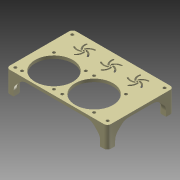
# Autodesk Inventor part: Tapa carcasa SAV
Saved by Autodesk Inventor 2014 (Build 180170000, 170)
## iProperties
Created: 2014-09-11
Part Number: Tapa carcasa SAV
Material: Nylon, molybdenum disulphide
Document SubType Name: Modeling
Designer: Rubén
Density: 1.13 g/cm^3
Appearance: Nylon 6
Mass: 26.3943 g
Surface Area: 167.072 cm^2
Volume: 23.3578 cm^3
Author: Rubén
Autodesk Inventor part; units mm, degrees
ref_plane "YZ Plane" through (0, 0, 0) normal (1, 0, 0) x (0, 1, 0)
ref_plane "XZ Plane" through (0, 0, 0) normal (0, 1, 0) x (-1, 0, 0)
ref_plane "XY Plane" through (0, 0, 0) normal (0, 0, 1) x (1, 0, 0)
sketch "Sketch1" plane through (0, 0, 0) normal (0, 1, 0) x (-1, 0, 0)
  line L0 (6.59, 3) -> (101.11, 3)
  line L1 (104.7, 6.59) -> (104.7, 66.18)
  line L2 (101.11, 69.77) -> (6.59, 69.77)
  line L3 (3, 66.18) -> (3, 6.59)
  arc A0 (6.59, 69.77) -> (3, 66.18) centre (6.59, 66.18) ccw
  arc A1 (104.7, 66.18) -> (101.11, 69.77) centre (101.11, 66.18) ccw
  arc A2 (101.11, 3) -> (104.7, 6.59) centre (101.11, 6.59) ccw
  arc A3 (3, 6.59) -> (6.59, 3) centre (6.59, 6.59) ccw
  line L4 (61.1, 41.9) -> (61.1, 62.5) construction
  line L5 (61.1, 41.9) -> (97.35, 41.9) construction
  line L6 (61.1, 41.9) -> (24.85, 41.9) construction
  line L7 (24.85, 41.9) -> (24.85, 62.5) construction
  line L8 (24.85, 62.5) -> (97.35, 62.5) construction
  line L9 (97.35, 62.5) -> (97.35, 41.9) construction
  line L10 (61.8884, 68.7185) -> (93.8884, 68.7185) construction
  line L11 (98.0634, 64.5435) -> (98.0634, 32.5435) construction
  line L12 (93.8884, 28.3685) -> (61.8884, 28.3685) construction
  line L13 (57.7134, 32.5435) -> (57.7134, 64.5435) construction
  line L14 (53.5384, 68.7185) -> (21.5384, 68.7185) construction
  line L15 (17.3634, 64.5435) -> (17.3634, 32.5435) construction
  line L16 (21.5384, 28.3685) -> (53.5384, 28.3685) construction
  circle A4 centre (21.538, 32.544) radius 1.5
  arc A5 (21.5384, 68.7185) -> (17.3634, 64.5435) centre (21.5384, 64.5435) ccw construction
  arc A6 (17.3634, 32.5435) -> (21.5384, 28.3685) centre (21.5384, 32.5435) ccw construction
  arc A7 (53.5384, 28.3685) -> (57.7134, 32.5435) centre (53.5384, 32.5435) ccw construction
  arc A8 (57.7134, 32.5435) -> (61.8884, 28.3685) centre (61.8884, 32.5435) ccw construction
  arc A9 (93.8884, 28.3685) -> (98.0634, 32.5435) centre (93.8884, 32.5435) ccw construction
  arc A10 (98.0634, 64.5435) -> (93.8884, 68.7185) centre (93.8884, 64.5435) ccw construction
  arc A11 (57.7134, 64.5435) -> (53.5384, 68.7185) centre (53.5384, 64.5435) ccw construction
  arc A12 (61.8884, 68.7185) -> (57.7134, 64.5435) centre (61.8884, 64.5435) ccw construction
  circle A13 centre (21.5384, 64.5435) radius 1.5
  circle A14 centre (61.8884, 64.5435) radius 1.5
  circle A15 centre (53.5384, 64.5435) radius 1.5
  circle A16 centre (93.8884, 64.5435) radius 1.5
  circle A17 centre (61.8884, 32.5435) radius 1.5
  circle A18 centre (53.5384, 32.5435) radius 1.5
  circle A19 centre (93.8884, 32.5435) radius 1.5
  circle A20 centre (37.5384, 48.5435) radius 19
  circle A21 centre (77.8884, 48.5435) radius 19
  circle A22 centre (53.85, 15.8218) radius 0.75
  arc A23 (58.578, 8.7134) -> (56.37, 16.3622) centre (50.85, 10.6256) ccw
  arc A24 (57.122, 9.0737) -> (55.33, 15.2814) centre (50.85, 10.6256) ccw
  arc A25 (57.122, 9.0737) -> (58.578, 8.7134) centre (57.85, 8.8936) ccw
  arc A26 (56.37, 16.3622) -> (55.33, 15.2814) centre (55.85, 15.8218) ccw
  circle A27 centre (80.75, 15.8218) radius 0.75
  arc A28 (85.478, 8.7134) -> (83.27, 16.3622) centre (77.75, 10.6256) ccw
  arc A29 (84.022, 9.0737) -> (82.23, 15.2814) centre (77.75, 10.6256) ccw
  arc A30 (84.022, 9.0737) -> (85.478, 8.7134) centre (84.75, 8.8936) ccw
  arc A31 (83.27, 16.3622) -> (82.23, 15.2814) centre (82.75, 15.8218) ccw
  arc A32 (88.9715, 18.1218) -> (81.0148, 18.3855) centre (84.7648, 11.3629) ccw
  arc A33 (88.1789, 16.8483) -> (81.7213, 17.0623) centre (84.7648, 11.3629) ccw
  arc A34 (81.0148, 18.3855) -> (81.7213, 17.0623) centre (81.368, 17.7239) ccw
  arc A35 (88.1789, 16.8483) -> (88.9715, 18.1218) centre (88.5752, 17.4851) ccw
  arc A36 (81.1031, 24.3516) -> (78.3936, 16.8658) centre (86.2313, 18.2622) ccw
  arc A37 (82.0693, 23.2043) -> (79.8703, 17.1289) centre (86.2313, 18.2622) ccw
  arc A38 (78.3936, 16.8658) -> (79.8703, 17.1289) centre (79.132, 16.9974) ccw
  arc A39 (82.0693, 23.2043) -> (81.1031, 24.3516) centre (81.5862, 23.778) ccw
  arc A40 (72.7468, 18.7935) -> (79.0289, 13.9033) centre (80.1228, 21.7889) ccw
  arc A41 (74.1365, 19.3579) -> (79.235, 15.3891) centre (80.1228, 21.7889) ccw
  arc A42 (79.0289, 13.9033) -> (79.235, 15.3891) centre (79.132, 14.6462) ccw
  arc A43 (74.1365, 19.3579) -> (72.7468, 18.7935) centre (73.4416, 19.0757) ccw
  arc A44 (75.4506, 9.1285) -> (82.0427, 13.5921) centre (74.8811, 17.0693) ccw
  arc A45 (75.3433, 10.6247) -> (80.6934, 14.2473) centre (74.8811, 17.0693) ccw
  arc A46 (82.0427, 13.5921) -> (80.6934, 14.2473) centre (81.368, 13.9197) ccw
  arc A47 (75.3433, 10.6247) -> (75.4506, 9.1285) centre (75.397, 9.8766) ccw
  circle A48 centre (26.95, 15.8218) radius 0.75
  arc A49 (31.678, 8.7134) -> (29.47, 16.3622) centre (23.95, 10.6256) ccw
  arc A50 (30.222, 9.0737) -> (28.43, 15.2814) centre (23.95, 10.6256) ccw
  arc A51 (30.222, 9.0737) -> (31.678, 8.7134) centre (30.95, 8.8936) ccw
  arc A52 (29.47, 16.3622) -> (28.43, 15.2814) centre (28.95, 15.8218) ccw
  arc A53 (35.1715, 18.1218) -> (27.2148, 18.3855) centre (30.9648, 11.3629) ccw
  arc A54 (34.3789, 16.8483) -> (27.9213, 17.0623) centre (30.9648, 11.3629) ccw
  arc A55 (27.2148, 18.3855) -> (27.9213, 17.0623) centre (27.568, 17.7239) ccw
  arc A56 (34.3789, 16.8483) -> (35.1715, 18.1218) centre (34.7752, 17.4851) ccw
  arc A57 (27.3031, 24.3516) -> (24.5936, 16.8658) centre (32.4313, 18.2622) ccw
  arc A58 (28.2693, 23.2043) -> (26.0703, 17.1289) centre (32.4313, 18.2622) ccw
  arc A59 (24.5936, 16.8658) -> (26.0703, 17.1289) centre (25.332, 16.9974) ccw
  arc A60 (28.2693, 23.2043) -> (27.3031, 24.3516) centre (27.7862, 23.778) ccw
  arc A61 (18.9468, 18.7935) -> (25.2289, 13.9033) centre (26.3228, 21.7889) ccw
  arc A62 (20.3365, 19.3579) -> (25.435, 15.3891) centre (26.3228, 21.7889) ccw
  arc A63 (25.2289, 13.9033) -> (25.435, 15.3891) centre (25.332, 14.6462) ccw
  arc A64 (20.3365, 19.3579) -> (18.9468, 18.7935) centre (19.6416, 19.0757) ccw
  arc A65 (21.6506, 9.1285) -> (28.2427, 13.5921) centre (21.0811, 17.0693) ccw
  arc A66 (21.5433, 10.6247) -> (26.8934, 14.2473) centre (21.0811, 17.0693) ccw
  arc A67 (28.2427, 13.5921) -> (26.8934, 14.2473) centre (27.568, 13.9197) ccw
  arc A68 (21.5433, 10.6247) -> (21.6506, 9.1285) centre (21.597, 9.8766) ccw
  circle A69 centre (53.85, 15.8218) radius 0.75
  arc A70 (58.578, 8.7134) -> (56.37, 16.3622) centre (50.85, 10.6256) ccw
  arc A71 (57.122, 9.0737) -> (55.33, 15.2814) centre (50.85, 10.6256) ccw
  arc A72 (57.122, 9.0737) -> (58.578, 8.7134) centre (57.85, 8.8936) ccw
  arc A73 (56.37, 16.3622) -> (55.33, 15.2814) centre (55.85, 15.8218) ccw
  arc A74 (62.0715, 18.1218) -> (54.1148, 18.3855) centre (57.8648, 11.3629) ccw
  arc A75 (61.2789, 16.8483) -> (54.8213, 17.0623) centre (57.8648, 11.3629) ccw
  arc A76 (54.1148, 18.3855) -> (54.8213, 17.0623) centre (54.468, 17.7239) ccw
  arc A77 (61.2789, 16.8483) -> (62.0715, 18.1218) centre (61.6752, 17.4851) ccw
  arc A78 (54.2031, 24.3516) -> (51.4936, 16.8658) centre (59.3313, 18.2622) ccw
  arc A79 (55.1693, 23.2043) -> (52.9703, 17.1289) centre (59.3313, 18.2622) ccw
  arc A80 (51.4936, 16.8658) -> (52.9703, 17.1289) centre (52.232, 16.9974) ccw
  arc A81 (55.1693, 23.2043) -> (54.2031, 24.3516) centre (54.6862, 23.778) ccw
  arc A82 (45.8468, 18.7935) -> (52.1289, 13.9033) centre (53.2228, 21.7889) ccw
  arc A83 (47.2365, 19.3579) -> (52.335, 15.3891) centre (53.2228, 21.7889) ccw
  arc A84 (52.1289, 13.9033) -> (52.335, 15.3891) centre (52.232, 14.6462) ccw
  arc A85 (47.2365, 19.3579) -> (45.8468, 18.7935) centre (46.5416, 19.0757) ccw
  arc A86 (48.5506, 9.1285) -> (55.1427, 13.5921) centre (47.9811, 17.0693) ccw
  arc A87 (48.4433, 10.6247) -> (53.7934, 14.2473) centre (47.9811, 17.0693) ccw
  arc A88 (55.1427, 13.5921) -> (53.7934, 14.2473) centre (54.468, 13.9197) ccw
  arc A89 (48.4433, 10.6247) -> (48.5506, 9.1285) centre (48.497, 9.8766) ccw
  circle A90 centre (7.495, 64.96) radius 1.5
  circle A91 centre (7.495, 7.81) radius 1.5
  circle A92 centre (100.205, 7.81) radius 1.5
  circle A93 centre (100.205, 64.96) radius 1.5
  line L17 (3, 36.385) -> (104.7, 36.385) construction
  line L18 (53.85, 3) -> (53.85, 69.77) construction
  point P0 (0, 0)
  point P1 (3, 3)
  point P2 (104.7, 3)
  point P3 (104.7, 69.77)
  point P4 (3, 69.77)
  point P5 (57.7134, 68.7185)
  point P6 (98.0634, 28.3685)
  point P7 (98.0634, 68.7185)
  point P8 (57.7134, 28.3685)
  point P9 (17.3634, 68.7185)
  point P10 (17.3634, 28.3685)
  point P11 (61.6752, 17.4851)
  point P12 (61.2789, 16.8483)
  point P13 (54.8213, 17.0623)
  point P14 (52.232, 16.9974)
  point P15 (59.3313, 18.2622)
  point P16 (52.9703, 17.1289)
  point P17 (45.8468, 18.7935)
  point P18 (47.2365, 19.3579)
  point P19 (52.1289, 13.9033)
  point P20 (48.497, 9.8766)
  point P21 (48.4433, 10.6247)
  point P22 (53.7934, 14.2473)
  dimension "d2" = 101.7
  dimension "d3" = 66.77
  dimension "d4" = 101.7
  dimension "d5" = 3.59
  dimension "d6" = 3.59
  dimension "d21" = 36.25
  dimension "d22" = 36.25
  dimension "d23" = 20.6
  dimension "d24" = 40.35
  dimension "d25" = 40.35
  dimension "d26" = 40.35
  dimension "d27" = 40.35
  dimension "d28" = 40.35
  dimension "d29" = 3
  dimension "d30" = 4.175
  dimension "d31" = 3
  dimension "d32" = 3
  dimension "d33" = 3
  dimension "d34" = 3
  dimension "d35" = 3
  dimension "d36" = 3
  dimension "d37" = 3
  dimension "d40" = 38
  dimension "d41" = 38
  dimension "d71" = 26.9
  dimension "d74" = 26.9
  dimension "d83" = 3
  dimension "d84" = 3
  dimension "d85" = 3
  dimension "d86" = 3
  dimension "d192" = 57.15
  dimension "d193" = 28.575
  dimension "d194" = 57.15
  dimension "d195" = 28.575
  dimension "d196" = 92.71
  dimension "d197" = 92.71
  dimension "d198" = 46.355
  dimension "d199" = 46.355
  constraints: 152 point on circle, 94 centre point, 38 end point, 28 tangent, 24 point on line, 9 equal radius, 8 perpendicular, 7 coincident, 5 midpoint, 4 equal length, 3 horizontal
  measures "d2" distance of point (3, 3) point (104.7, 3)
  measures "d3" distance of point (104.7, 3) point (104.7, 69.77)
  measures "d4" distance of point (104.7, 69.77) point (3, 69.77)
  measures "d5" radius of A0
  measures "d6" radius of A1
  measures "d21" distance of L4.start L5.end
  measures "d22" distance of L4.start L6.end
  measures "d23" distance of L6.end L7.end
  measures "d24" distance of point (98.063, 28.369) point (57.713, 28.369)
  measures "d25" distance of point (98.063, 68.719) point (98.063, 28.369)
  measures "d26" distance of point (57.713, 68.719) point (17.363, 68.719)
  measures "d27" distance of point (17.363, 68.719) point (17.363, 28.369)
  measures "d28" distance of point (17.363, 28.369) point (57.713, 28.369)
  measures "d29" diameter of A4
  measures "d30" radius of A5
  measures "d31" diameter of A13
  measures "d32" diameter of A14
  measures "d33" diameter of A15
  measures "d34" diameter of A16
  measures "d35" diameter of A17
  measures "d36" diameter of A18
  measures "d37" diameter of A19
  measures "d40" diameter of A20
  measures "d41" diameter of A21
  measures "d71" distance of point (59.331, 18.262) A36.centre
  measures "d74" distance of point (59.331, 18.262) A57.centre
  measures "d83" diameter of A90
  measures "d84" diameter of A91
  measures "d85" diameter of A92
  measures "d86" diameter of A93
  measures "d192" distance of A91.centre A90.centre
  measures "d193" distance from line of L17 A91.centre
  measures "d194" distance of A93.centre A92.centre
  measures "d195" distance from line of L17 A92.centre
  measures "d196" distance of A93.centre A90.centre
  measures "d197" distance of A92.centre A91.centre
  measures "d198" distance from line of L18 A91.centre
  measures "d199" distance from line of L18 A90.centre
extrude "Extrusion3" add sketch "Sketch1" along normal blind 3
sketch "Sketch5" plane through (0, 0, 0) normal (0, -1, 0) x (1, 0, 0)
  circle A0 centre (-100.205, 64.96) radius 1.5 projected
  circle A1 centre (-100.205, 7.81) radius 1.5 projected
  line L0 (-6.59, 69.77) -> (-101.11, 69.77) projected
  line L1 (-104.7, 66.18) -> (-104.7, 6.59) projected
  line L2 (-101.11, 3) -> (-6.59, 3) projected
  line L3 (-3, 6.59) -> (-3, 66.18) projected
  arc A2 (-101.11, 69.77) -> (-104.7, 66.18) centre (-101.11, 66.18) ccw projected
  arc A3 (-104.7, 6.59) -> (-101.11, 3) centre (-101.11, 6.59) ccw projected
  arc A4 (-6.59, 3) -> (-3, 6.59) centre (-6.59, 6.59) ccw projected
  arc A5 (-3, 66.18) -> (-6.59, 69.77) centre (-6.59, 66.18) ccw projected
  line L4 (-97.205, 69.77) -> (-101.11, 69.77)
  line L5 (-104.7, 10.81) -> (-104.7, 6.59)
  line L6 (-101.11, 3) -> (-97.205, 3)
  line L7 (-10.495, 3) -> (-6.59, 3)
  line L8 (-3, 6.59) -> (-3, 10.81)
  line L9 (-10.495, 69.77) -> (-6.59, 69.77)
  line L10 (-3, 66.18) -> (-3, 61.96)
  arc A6 (-3, 66.18) -> (-6.59, 69.77) centre (-6.59, 66.18) ccw
  arc A7 (-6.59, 3) -> (-3, 6.59) centre (-6.59, 6.59) ccw
  arc A8 (-104.7, 6.59) -> (-101.11, 3) centre (-101.11, 6.59) ccw
  arc A9 (-101.11, 69.77) -> (-104.7, 66.18) centre (-101.11, 66.18) ccw
  circle A10 centre (-7.495, 7.81) radius 1.5
  circle A11 centre (-7.495, 64.96) radius 1.5
  circle A12 centre (-100.205, 7.81) radius 1.5
  circle A13 centre (-100.205, 64.96) radius 1.5
  arc A14 (-97.205, 7.81) -> (-100.205, 10.81) centre (-100.205, 7.81) ccw
  line L11 (-97.205, 7.81) -> (-97.205, 3)
  line L12 (-100.205, 10.81) -> (-104.7, 10.81)
  arc A15 (-100.205, 61.96) -> (-97.205, 64.96) centre (-100.205, 64.96) ccw
  arc A16 (-10.495, 64.96) -> (-7.495, 61.96) centre (-7.495, 64.96) ccw
  arc A17 (-7.495, 10.81) -> (-10.495, 7.81) centre (-7.495, 7.81) ccw
  line L13 (-7.495, 10.81) -> (-3, 10.81)
  line L14 (-10.495, 7.81) -> (-10.495, 3)
  line L15 (-97.205, 64.96) -> (-97.205, 69.77)
  line L16 (-7.495, 61.96) -> (-3, 61.96)
  line L17 (-10.495, 64.96) -> (-10.495, 69.77)
  circle A18 centre (-7.495, 7.81) radius 1.5 projected
  circle A19 centre (-7.495, 64.96) radius 1.5 projected
  line L18 (-100.205, 61.96) -> (-104.7, 61.96)
  line L19 (-104.7, 66.18) -> (-104.7, 61.96)
  point P0 (-3, 63.52)
  point P1 (-9.25, 69.77)
  point P2 (-104.7, 9.25)
  point P3 (-98.45, 3)
  point P4 (-98.45, 69.77)
  point P5 (-3, 9.25)
  point P6 (-9.25, 3)
  dimension "d142" = 3
  dimension "d143" = 3
  dimension "d144" = 3
  dimension "d145" = 3
  dimension "d146" = 6
  dimension "d147" = 6
  dimension "d148" = 6
  dimension "d149" = 6
  constraints: 32 end point, 22 point on circle, 22 point on line, 12 centre point, 12 coincident, 11 perpendicular, 10 tangent, 3 collinear
  measures "d142" diameter of A10
  measures "d143" diameter of A11
  measures "d144" diameter of A12
  measures "d145" diameter of A13
  measures "d146" diameter of A14
  measures "d147" diameter of A15
  measures "d148" diameter of A16
  measures "d149" diameter of A17
extrude "Extrusion6" add sketch "Sketch5" along normal blind 18.4 contours A5 L3 L16 A16 L17 L0 | L15 A15 L18 L1 A2 L0 | L3 A4 L2 L14 A17 L13 | L12 A14 L11 L2 A3 L1
sketch "Sketch6" plane through (-101.11, 3, 69.77) normal (0, 0, 1) x (1, 0, 0)
  line L0 (6.8339, -9.2711) -> (10.1761, -5.9289)
  arc A0 (17.2471, -3) -> (10.1761, -5.9289) centre (17.2471, -13) ccw
  arc A1 (6.8339, -9.2711) -> (3.905, -16.3421) centre (13.905, -16.3421) ccw
  line L1 (3.905, -3) -> (3.905, -16.3421)
  line L2 (3.905, -3) -> (17.2471, -3)
  line L3 (94.52, -21.4) -> (90.615, -21.4) projected
  line L4 (47.42, -3) -> (47.42, -21.4) construction
  line L5 (88.0061, -9.2711) -> (84.6639, -5.9289)
  arc A2 (84.6639, -5.9289) -> (77.5928, -3) centre (77.5928, -13) ccw
  arc A3 (90.935, -16.3421) -> (88.0061, -9.2711) centre (80.935, -16.3421) ccw
  line L6 (90.935, -3) -> (90.935, -16.3421)
  line L7 (90.935, -3) -> (77.5928, -3)
  point P0 (91.86, -21.4)
  point P1 (101.11, -3)
  point P2 (13.105, -3)
  point P3 (94.52, -3)
  point P4 (0, -3)
  point P5 (3.905, -3)
  point P6 (91.63, -21.4)
  point P7 (81.735, -3)
  point P8 (90.935, -3)
  dimension "d94" = 10
  dimension "d95" = 10
  constraints: 14 end point, 9 symmetric about line, 8 point on circle, 4 centre point, 4 tangent, 2 point on line, 1 perpendicular, 2 other
  measures "d94" radius of A0
  measures "d95" radius of A1
extrude "Extrusion7" add sketch "Sketch6" against normal blind 2.8
sketch "Sketch7" plane through (-6.59, 3, 3) normal (0, 0, -1) x (-1, 0, 0)
  line L0 (90.615, -3) -> (3.905, -3) projected
  line L1 (6.8339, -9.2711) -> (10.1761, -5.9289)
  arc A0 (17.2471, -3) -> (10.1761, -5.9289) centre (17.2471, -13) ccw
  arc A1 (6.8339, -9.2711) -> (3.905, -16.3421) centre (13.905, -16.3421) ccw
  line L2 (3.905, -3) -> (3.905, -16.3421)
  line L3 (3.905, -3) -> (17.2471, -3)
  line L4 (47.26, -3) -> (47.26, -21.4) construction
  line L5 (87.6861, -9.2711) -> (84.3439, -5.9289)
  arc A2 (84.3439, -5.9289) -> (77.2729, -3) centre (77.2729, -13) ccw
  arc A3 (90.615, -16.3421) -> (87.6861, -9.2711) centre (80.615, -16.3421) ccw
  line L6 (90.615, -3) -> (90.615, -16.3421)
  line L7 (90.615, -3) -> (77.2729, -3)
  point P0 (2.66, -3)
  point P1 (-6.59, -3)
  point P2 (94.52, -3)
  point P3 (0, -3)
  constraints: 14 end point, 10 point on circle, 9 symmetric about line, 4 centre point, 3 tangent, 1 collinear, 1 equal radius, 1 midpoint, 1 perpendicular, 2 other
extrude "Extrusion8" add sketch "Sketch7" against normal blind 4.81
sketch "Sketch8" plane through (-104.7, 3, 6.59) normal (-1, 0, 0) x (0, 0, 1)
  line L0 (55.37, -3) -> (4.22, -3) projected
  line L1 (59.59, -21.4) -> (0, -21.4) projected
  line L2 (29.795, -3) -> (29.795, -21.4) construction
  line L3 (7.1489, -9.2711) -> (10.4911, -5.9289)
  arc A0 (17.5621, -3) -> (10.4911, -5.9289) centre (17.5621, -13) ccw
  arc A1 (7.1489, -9.2711) -> (4.22, -16.3421) centre (14.22, -16.3421) ccw
  line L4 (4.22, -16.3421) -> (4.22, -3)
  line L5 (17.5621, -3) -> (4.22, -3)
  line L6 (52.4411, -9.2711) -> (49.0989, -5.9289)
  arc A2 (49.0989, -5.9289) -> (42.0279, -3) centre (42.0279, -13) ccw
  arc A3 (55.37, -16.3421) -> (52.4411, -9.2711) centre (45.37, -16.3421) ccw
  line L7 (55.37, -16.3421) -> (55.37, -3)
  line L8 (42.0279, -3) -> (55.37, -3)
  point P0 (56.93, -21.4)
  point P1 (-6.59, -3)
  point P2 (59.59, -3)
  point P3 (0, -3)
  point P4 (55.37, -3)
  constraints: 14 end point, 8 point on circle, 8 symmetric about line, 4 centre point, 4 tangent, 2 perpendicular, 1 equal radius, 1 midpoint, 2 other
extrude "Extrusion9" add sketch "Sketch8" against normal blind 4.495
sketch "Sketch9" plane through (-3, 3, 66.18) normal (1, 0, 0) x (0, 0, -1)
  line L0 (55.37, -3) -> (4.22, -3) projected
  line L1 (29.795, -3) -> (29.795, -21.4) construction
  line L2 (7.1489, -9.2711) -> (10.4911, -5.9289)
  arc A0 (17.5621, -3) -> (10.4911, -5.9289) centre (17.5621, -13) ccw
  arc A1 (7.1489, -9.2711) -> (4.22, -16.3421) centre (14.22, -16.3421) ccw
  line L3 (17.5621, -3) -> (4.22, -3)
  line L4 (4.22, -16.3421) -> (4.22, -3)
  line L5 (52.4411, -9.2711) -> (49.0989, -5.9289)
  arc A2 (49.0989, -5.9289) -> (42.0279, -3) centre (42.0279, -13) ccw
  arc A3 (55.37, -16.3421) -> (52.4411, -9.2711) centre (45.37, -16.3421) ccw
  line L6 (42.0279, -3) -> (55.37, -3)
  line L7 (55.37, -16.3421) -> (55.37, -3)
  point P0 (66.18, -3)
  point P1 (13.42, -3)
  point P2 (59.59, -3)
  point P3 (0, -3)
  point P4 (46.17, -3)
  constraints: 14 end point, 9 symmetric about line, 8 point on circle, 4 centre point, 4 tangent, 2 point on line, 1 collinear, 1 equal radius, 1 midpoint, 2 other
extrude "Extrusion10" add sketch "Sketch9" against normal blind 4.495
sketch "Sketch14" plane through (0, -18.4, 0) normal (0, -1, 0) x (1, 0, 0)
  circle A0 centre (-7.495, 64.96) radius 1.5 projected
  arc A1 (-10.495, 64.96) -> (-7.495, 61.96) centre (-7.495, 64.96) ccw projected
  circle A2 centre (-7.495, 64.96) radius 1.65
  point P0 (0, 0)
  dimension "d159" = 3.3
  constraints: 1 centre point, 1 coincident
  measures "d159" diameter of A2
hole "Hole5" at (-7.495, -18.4, 64.96) direction (0, 1, 0) diameter 3.4 depth 17 tip angle 118
sketch "Sketch15" plane through (0, -18.4, 0) normal (0, -1, 0) x (1, 0, 0)
  arc A0 (-98.705, 7.81) -> (-98.705, 7.81) centre (-100.205, 7.81) ccw projected
  arc A1 (-97.205, 7.81) -> (-100.205, 10.81) centre (-100.205, 7.81) ccw projected
  circle A2 centre (-100.205, 7.81) radius 1.65
  point P0 (0, 0)
  dimension "d167" = 3.3
  constraints: 1 centre point, 1 coincident
  measures "d167" diameter of A2
hole "Hole6" at (-100.205, -18.4, 7.81) direction (0, 1, 0) diameter 3.4 depth 17 tip angle 118
sketch "Sketch16" plane through (0, -18.4, 0) normal (0, -1, 0) x (1, 0, 0)
  circle A0 centre (-7.495, 7.81) radius 1.5 projected
  arc A1 (-7.495, 10.81) -> (-10.495, 7.81) centre (-7.495, 7.81) ccw projected
  circle A2 centre (-7.495, 7.81) radius 1.65
  point P0 (0, 0)
  dimension "d175" = 3.3
  constraints: 1 centre point, 1 coincident
  measures "d175" diameter of A2
hole "Hole7" at (-7.495, -18.4, 7.81) direction (0, 1, 0) diameter 3.4 depth 17 tip angle 118
sketch "Sketch17" plane through (0, -18.4, 0) normal (0, -1, 0) x (1, 0, 0)
  arc A0 (-98.705, 64.96) -> (-98.705, 64.96) centre (-100.205, 64.96) ccw projected
  arc A1 (-100.205, 61.96) -> (-97.205, 64.96) centre (-100.205, 64.96) ccw projected
  circle A2 centre (-100.205, 64.96) radius 1.65
  point P0 (0, 0)
  dimension "d183" = 3.3
  constraints: 1 centre point, 1 coincident
  measures "d183" diameter of A2
hole "Hole8" at (-100.205, -18.4, 64.96) direction (0, 1, 0) diameter 3.4 depth 17 tip angle 118
body "Solid3"
